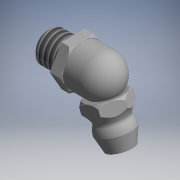
# Autodesk Inventor part: hsr_ftht_B-M6F_grease_nipple_joint
Saved by Autodesk Inventor 2017.3 (Build 213256000, 256)
## iProperties
Part Number: hsr_ftht_B-M6F_grease_nipple_joint
Material: Generic
Catalog Web Link: www.cadenas.de
Description: HSR_ftht Grease Nipple Joint-Grease Nipple Joint
Vendor: THK
Document SubType Name: Modeling
Designer: partserver
Manufacturer: THK
Mass: 0.801446 g
Surface Area: 5.68367 cm^2
Volume: 0.801446 cm^3
Density: 1 g/cm^3
Appearance: PSOLRGB-192-192-192
Category: PARTsolutions
Company: THK
Title: hsr_ftht_B-M6F_grease_nipple_joint
Author: Cadenas PARTsolutions
Comments: Grease Nipple Joint
PSOL_IDENT_0: {$CADENAS_DATA\23d-libs\thk\linear_motion_systems\lm_guide\lm_guide\lm_guide_hsr\four_taped_hole_typ
PSOL_IDENT_1: e\hsr_ftht_grease_nipple_joint.prj},232 {VTYP=3D},{NB=hsr_ftht_B-M6F_grease_nipple_joint},{LINA=hsr_
PSOL_IDENT_2: ftht_B-M6F_grease_nipple_joint},{NN=HSR_ftht Grease Nipple Joint},{DATE=08.06.2021 00:57:46},{GEOMDA
PSOL_IDENT_3: TE=02.02.2021 11:34:29},{VERSION=},{LINEID=10},{WBVAR=MN},{WBNUMERIC=}  {NB=hsr_ftht_B-M6F_grease_ni
PSOL_IDENT_4: pple_joint},{LINA=hsr_ftht_B-M6F_grease_nipple_joint},{KT=DUMMY},{MN=B-M6F},{E=11.6},{A=5},{B=3},{C=
PSOL_IDENT_5: 8},{X=1},{Y=2},{NOTE=MIN}
NB: hsr_ftht_B-M6F_grease_nipple_joint
NN: HSR_ftht Grease Nipple Joint
NT: Grease Nipple Joint
NBSYN: hsr_ftht_$MN._grease_nipple_joint
LINA: hsr_ftht_B-M6F_grease_nipple_joint
CATALOG: THK
MN: B-M6F
NOTE: 0
SUPPLIER: THK
ARTICLENO: hsr_ftht_B-M6F_grease_nipple_joint
BOMINFO: hsr_ftht_B-M6F_grease_nipple_joint
CREATOR: CADENAS GmbH
Autodesk Inventor part; units mm, degrees
sketch "Sketch_1" plane through (0, 0, 0) normal (0, 0, 1) x (1, 0, 0)
  line L0 (5, 0) -> (0, 0)
  line L1 (0, 0) -> (0, 3)
  line L2 (0, 3) -> (4.3865, 3)
  line L3 (4.3865, 3) -> (5, 2.3865)
  line L4 (5, 2.3865) -> (5, 0)
  line L5 (5, 0) -> (0, 0)
  constraints: 12 end point
revolve "Revolution1" add sketch "Sketch_1" angle 360 about axis through (5, 0, 0) along (1, 0, 0)
thread "Thread1" size "M6x1" class "6g" standard "ISO Metric profile" length 3.8434
sketch "Sketch_5" plane through (0, 0, 0) normal (0, 0, 1) x (1, 0, 0)
  line L0 (0, 0) -> (-5.3, 0)
  arc A0 (-5.3, 4) -> (-9.3, 0) centre (-5.3, 0) ccw
  line L1 (-5.3, 4) -> (-2, 4)
  line L2 (-2, 4) -> (-2, 4.12)
  line L3 (-2, 4.12) -> (-1.5, 4.62)
  line L4 (-1.5, 4.62) -> (0, 4.62)
  line L5 (0, 4.62) -> (0, 0)
  line L6 (0, 0) -> (-9.3, 0)
  constraints: 14 end point, 2 point on circle, 1 centre point
revolve "Revolution2" add sketch "Sketch_5" angle 360 about axis through (0, 0, 0) along (1, 0, 0)
sketch "Sketch_13" plane through (0, 0, 0) normal (1, 0, 0) x (0, 1, 0)
  line L0 (16, 16) -> (-16, 16)
  line L1 (-16, 16) -> (-16, -16)
  line L2 (-16, -16) -> (16, -16)
  line L3 (16, -16) -> (16, 16)
  line L4 (-2.3094, 4) -> (-4.6188, 0)
  line L5 (-4.6188, 0) -> (-2.3094, -4)
  line L6 (-2.3094, -4) -> (2.3094, -4)
  line L7 (2.3094, -4) -> (4.6188, 0)
  line L8 (4.6188, 0) -> (2.3094, 4)
  line L9 (2.3094, 4) -> (-2.3094, 4)
  constraints: 20 end point
extrude "Extrusion1" cut sketch "Sketch_13" against normal blind 5
sketch "Sketch_17" plane through (-5.1495, 0, 0) normal (0.9271839, 0, 0.3746066) x (0.3746066, 0, -0.9271839)
  line L0 (-11.22, 0) -> (-3.12, 0)
  line L1 (-3.12, 0) -> (-3.12, -3.4448)
  line L2 (-3.12, -3.4448) -> (-3.7352, -4.06)
  line L3 (-3.7352, -4.06) -> (-4.852, -4.06)
  arc A0 (-4.852, -4.06) -> (-6.3637, -2.9706) centre (-9.0732, -8.324) ccw
  arc A1 (-6.3637, -2.9706) -> (-7.076, -2.9655) centre (-6.725, -3.6844) ccw
  arc A2 (-8.5237, -3.3) -> (-7.076, -2.9655) centre (-8.5237, 0) ccw
  line L4 (-8.5237, -3.3) -> (-11.22, -2.4239)
  line L5 (-11.22, -2.4239) -> (-11.22, -1.1171)
  arc A3 (-11.6032, 0) -> (-11.22, -1.1171) centre (-9.7832, 0) ccw
  line L6 (-11.6032, 0) -> (-3.12, 0)
  constraints: 14 end point, 8 point on circle, 4 centre point
revolve "Revolution3" add sketch "Sketch_17" angle 360 about axis through (-9.3526, 0, 10.403) along (-0.3746066, 0, 0.9271839)
sketch "Sketch_18" plane through (-6.337, 0, 2.9392) normal (0.3746066, 0, -0.9271839) x (-0.9271839, 0, -0.3746066)
  line L0 (-7, 7) -> (-7, -7)
  line L1 (-7, -7) -> (7, -7)
  line L2 (7, -7) -> (7, 7)
  line L3 (7, 7) -> (-7, 7)
  line L4 (-4.0415, 0) -> (-2.0207, -3.5)
  line L5 (-2.0207, -3.5) -> (2.0207, -3.5)
  line L6 (2.0207, -3.5) -> (4.0415, 0)
  line L7 (4.0415, 0) -> (2.0207, 3.5)
  line L8 (2.0207, 3.5) -> (-2.0207, 3.5)
  line L9 (-2.0207, 3.5) -> (-4.0415, 0)
  constraints: 20 end point
extrude "Extrusion2" cut sketch "Sketch_18" against normal blind 2.5
ref_plane "n_j_XY" through (0, 0, 0) normal (1, 0, 0) x (0, 0, -1)
ref_plane "n_j_YZ" through (0, 0, 0) normal (0, 0, -1) x (0, 1, 0)
ref_plane "n_j_ZX" through (0, 0, 0) normal (0, 1, 0) x (1, 0, 0)
body "Solid1"
